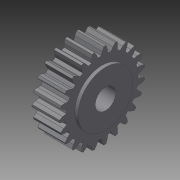
# Autodesk Inventor part: M-0.5 Zb-4mm M-0.7 Zb-5mm mN 21102300
Saved by Autodesk Inventor 2017.3 (Build 213256000, 256)
## iProperties
Category: PARTsolutions
Company: MAEDLER
Created: 2018-08-16
Part Number: M-0.5 Zb-4mm M-0.7 Zb-5mm mN 21102300
Material: Generic
Catalog Web Link: www.cadenas.de
Description: M-0.5 Zb-4mm M-0.7 Zb-5mm mN-Spur Gears, Steel, Module 0.5 and 0,7
Vendor: MAEDLER
Document SubType Name: Modeling
Designer: psadmin
Manufacturer: MAEDLER
Mass: 4 g
Surface Area: 6.38111 cm^2
Volume: 0.554317 cm^3
Density: 1 g/cm^3
Appearance: PSOLRGB-175-175-175
PSOL_IDENT_0: {$CADENAS_DATA\23d-libs\maedler\antriebselemente\stirnzahnraeder\stirnzahnraeder_stahl\modul_0.5_und
PSOL_IDENT_1: _0.7\m-0.5_zb-4mm_m-0.7_zb-5mm_mn.prj},237 {VTYP=3D},{NB=M-0.5 Zb-4mm M-0.7 Zb-5mm mN 21102300},{LIN
PSOL_IDENT_2: A=M-0.5 Zb-4mm M-0.7 Zb-5mm mN 21102300},{NN=M-0.5 Zb-4mm M-0.7 Zb-5mm mN},{DATE=27.10.2015 07:21:56
PSOL_IDENT_3: },{GEOMDATE=11.05.2009 09:51:00},{VERSION=},{LINEID=130},{WBVAR=},{WBNUMERIC=}  {NB=M-0.5 Zb-4mm M-0
PSOL_IDENT_4: .7 Zb-5mm mN 21102300},{LINA=M-0.5 Zb-4mm M-0.7 Zb-5mm mN 21102300},{KT=DUMMY},{ARTNR=21102300},{WST=
PSOL_IDENT_5: 11SMnPb30},{M=0.5},{Z=23},{PDF=PDF Katalogseite},{B1=4.0},{DA=12.50},{D=11.50},{NL=4},{ND=8},{B=3},{
PSOL_IDENT_6: MD=3.0},{GEW=4.000}
NN: M-0.5 Zb-4mm M-0.7 Zb-5mm mN
NT: Spur Gears, Steel, Module 0.5 and 0,7
NB: M-0.5 Zb-4mm M-0.7 Zb-5mm mN 21102300
NBSYN: M-0.5 Zb-4mm M-0.7 Zb-5mm mN $ARTNR.
LINA: M-0.5 Zb-4mm M-0.7 Zb-5mm mN 21102300
ARTNR: 21102300
WST: 11SMnPb30
M: 0.5
Z: 23
PDF: PDF Katalogseite
B1: 4
DA: 12.5
D: 11.5
NL: 4
ND: 8
B: 3
MD: 3
GEW: 4
SUPPLIER: MAEDLER
ARTICLENO: M-0.5 Zb-4mm M-0.7 Zb-5mm mN 21102300
BOMINFO: M-0.5 Zb-4mm M-0.7 Zb-5mm mN 21102300
CREATOR: CADENAS GmbH
Title: M-0.5 Zb-4mm M-0.7 Zb-5mm mN 21102300
Author: Cadenas PARTsolutions
Comments: Spur Gears, Steel, Module 0.5 and 0,7
Autodesk Inventor part; units mm, degrees
ref_plane "YZ Plane" through (0, 0, 0) normal (1, 0, 0) x (0, 1, 0)
ref_plane "XZ Plane" through (0, 0, 0) normal (0, 1, 0) x (-1, 0, 0)
ref_plane "XY Plane" through (0, 0, 0) normal (0, 0, 1) x (1, 0, 0)
sketch "Skizze_1" plane through (0, 0, 0) normal (1, 0, 0) x (0, 1, 0)
  line L0 (0.2601, 6.2446) -> (0.0251, 5.7499)
  line L1 (0.0251, 5.7499) -> (-0.1195, 5.2486)
  arc A0 (-0.1195, 5.2486) -> (-0.5963, 5.216) centre (0, 0) ccw
  line L2 (-0.5963, 5.216) -> (-0.8078, 5.693)
  line L3 (-0.8078, 5.693) -> (-1.108, 6.151)
  arc A1 (-1.108, 6.151) -> (-1.4343, 6.0832) centre (0, 0) ccw
  line L4 (-1.4343, 6.0832) -> (-1.5272, 5.5435)
  line L5 (-1.5272, 5.5435) -> (-1.5311, 5.0218)
  arc A2 (-1.5311, 5.0218) -> (-1.9815, 4.8617) centre (0, 0) ccw
  line L6 (-1.9815, 4.8617) -> (-2.3138, 5.2639)
  line L7 (-2.3138, 5.2639) -> (-2.7264, 5.624)
  arc A3 (-2.7264, 5.624) -> (-3.0224, 5.4706) centre (0, 0) ccw
  line L8 (-3.0224, 5.4706) -> (-2.9662, 4.9259)
  line L9 (-2.9662, 4.9259) -> (-2.8292, 4.4224)
  arc A4 (-2.8292, 4.4224) -> (-3.2197, 4.1468) centre (0, 0) ccw
  line L10 (-3.2197, 4.1468) -> (-3.6482, 4.4445)
  line L11 (-3.6482, 4.4445) -> (-4.1426, 4.6799)
  arc A5 (-4.1426, 4.6799) -> (-4.3862, 4.4523) centre (0, 0) ccw
  line L12 (-4.3862, 4.4523) -> (-4.1852, 3.943)
  line L13 (-4.1852, 3.943) -> (-3.9175, 3.4951)
  arc A6 (-3.9175, 3.4951) -> (-4.2191, 3.1244) centre (0, 0) ccw
  line L14 (-4.2191, 3.1244) -> (-4.712, 3.2954)
  line L15 (-4.712, 3.2954) -> (-5.2516, 3.3886)
  arc A7 (-5.2516, 3.3886) -> (-5.4248, 3.1038) centre (0, 0) ccw
  line L16 (-5.4248, 3.1038) -> (-5.0938, 2.6676)
  line L17 (-5.0938, 2.6676) -> (-4.7152, 2.3086)
  arc A8 (-4.7152, 2.3086) -> (-4.9056, 1.8703) centre (0, 0) ccw
  line L18 (-4.9056, 1.8703) -> (-5.4263, 1.9019)
  line L19 (-5.4263, 1.9019) -> (-5.9711, 1.8461)
  arc A9 (-5.9711, 1.8461) -> (-6.0611, 1.5251) centre (0, 0) ccw
  line L20 (-6.0611, 1.5251) -> (-5.6246, 1.1944)
  line L21 (-5.6246, 1.1944) -> (-5.1632, 0.9509)
  arc A10 (-5.1632, 0.9509) -> (-5.2282, 0.4774) centre (0, 0) ccw
  line L22 (-5.2282, 0.4774) -> (-5.7383, 0.3674)
  line L23 (-5.7383, 0.3674) -> (-6.2478, 0.1667)
  arc A11 (-6.2478, 0.1667) -> (-6.2478, -0.1667) centre (0, 0) ccw
  line L24 (-6.2478, -0.1667) -> (-5.7383, -0.3674)
  line L25 (-5.7383, -0.3674) -> (-5.2282, -0.4774)
  arc A12 (-5.2282, -0.4774) -> (-5.1632, -0.9509) centre (0, 0) ccw
  line L26 (-5.1632, -0.9509) -> (-5.6246, -1.1944)
  line L27 (-5.6246, -1.1944) -> (-6.0611, -1.5251)
  arc A13 (-6.0611, -1.5251) -> (-5.9711, -1.8461) centre (0, 0) ccw
  line L28 (-5.9711, -1.8461) -> (-5.4263, -1.9019)
  line L29 (-5.4263, -1.9019) -> (-4.9056, -1.8703)
  arc A14 (-4.9056, -1.8703) -> (-4.7152, -2.3086) centre (0, 0) ccw
  line L30 (-4.7152, -2.3086) -> (-5.0938, -2.6676)
  line L31 (-5.0938, -2.6676) -> (-5.4248, -3.1038)
  arc A15 (-5.4248, -3.1038) -> (-5.2516, -3.3886) centre (0, 0) ccw
  line L32 (-5.2516, -3.3886) -> (-4.712, -3.2954)
  line L33 (-4.712, -3.2954) -> (-4.2191, -3.1244)
  arc A16 (-4.2191, -3.1244) -> (-3.9175, -3.4951) centre (0, 0) ccw
  line L34 (-3.9175, -3.4951) -> (-4.1852, -3.943)
  line L35 (-4.1852, -3.943) -> (-4.3862, -4.4523)
  arc A17 (-4.3862, -4.4523) -> (-4.1426, -4.6799) centre (0, 0) ccw
  line L36 (-4.1426, -4.6799) -> (-3.6482, -4.4445)
  line L37 (-3.6482, -4.4445) -> (-3.2197, -4.1468)
  arc A18 (-3.2197, -4.1468) -> (-2.8292, -4.4224) centre (0, 0) ccw
  line L38 (-2.8292, -4.4224) -> (-2.9662, -4.9259)
  line L39 (-2.9662, -4.9259) -> (-3.0224, -5.4706)
  arc A19 (-3.0224, -5.4706) -> (-2.7264, -5.624) centre (0, 0) ccw
  line L40 (-2.7264, -5.624) -> (-2.3138, -5.2639)
  line L41 (-2.3138, -5.2639) -> (-1.9815, -4.8617)
  arc A20 (-1.9815, -4.8617) -> (-1.5311, -5.0218) centre (0, 0) ccw
  line L42 (-1.5311, -5.0218) -> (-1.5272, -5.5435)
  line L43 (-1.5272, -5.5435) -> (-1.4343, -6.0832)
  arc A21 (-1.4343, -6.0832) -> (-1.108, -6.151) centre (0, 0) ccw
  line L44 (-1.108, -6.151) -> (-0.8078, -5.693)
  line L45 (-0.8078, -5.693) -> (-0.5963, -5.216)
  arc A22 (-0.5963, -5.216) -> (-0.1195, -5.2486) centre (0, 0) ccw
  line L46 (-0.1195, -5.2486) -> (0.0251, -5.7499)
  line L47 (0.0251, -5.7499) -> (0.2601, -6.2446)
  arc A23 (0.2601, -6.2446) -> (0.5926, -6.2218) centre (0, 0) ccw
  line L48 (0.5926, -6.2218) -> (0.7581, -5.6998)
  line L49 (0.7581, -5.6998) -> (0.8331, -5.1835)
  arc A24 (0.8331, -5.1835) -> (1.301, -5.0862) centre (0, 0) ccw
  line L50 (1.301, -5.0862) -> (1.5755, -5.53)
  line L51 (1.5755, -5.53) -> (1.9352, -5.9428)
  arc A25 (1.9352, -5.9428) -> (2.2493, -5.8312) centre (0, 0) ccw
  line L52 (2.2493, -5.8312) -> (2.2678, -5.2839)
  line L53 (2.2678, -5.2839) -> (2.2007, -4.7665)
  arc A26 (2.2007, -4.7665) -> (2.625, -4.5466) centre (0, 0) ccw
  line L54 (2.625, -4.5466) -> (3.009, -4.8998)
  line L55 (3.009, -4.8998) -> (3.4668, -5.2004)
  arc A27 (3.4668, -5.2004) -> (3.7391, -5.0081) centre (0, 0) ccw
  line L56 (3.7391, -5.0081) -> (3.6093, -4.4761)
  line L57 (3.6093, -4.4761) -> (3.4051, -3.996)
  arc A28 (3.4051, -3.996) -> (3.7543, -3.6698) centre (0, 0) ccw
  line L58 (3.7543, -3.6698) -> (4.2194, -3.9063)
  line L59 (4.2194, -3.9063) -> (4.7413, -4.0722)
  arc A29 (4.7413, -4.0722) -> (4.9517, -3.8136) centre (0, 0) ccw
  line L60 (4.9517, -3.8136) -> (4.6831, -3.3364)
  line L61 (4.6831, -3.3364) -> (4.3569, -2.9292)
  arc A30 (4.3569, -2.9292) -> (4.6052, -2.5208) centre (0, 0) ccw
  line L62 (4.6052, -2.5208) -> (5.1168, -2.6231)
  line L63 (5.1168, -2.6231) -> (5.6641, -2.642)
  arc A31 (5.6641, -2.642) -> (5.7969, -2.3363) centre (0, 0) ccw
  line L64 (5.7969, -2.3363) -> (5.4096, -1.9492)
  line L65 (5.4096, -1.9492) -> (4.9856, -1.6451)
  arc A32 (4.9856, -1.6451) -> (5.1145, -1.1849) centre (0, 0) ccw
  line L66 (5.1145, -1.1849) -> (5.6348, -1.1453)
  line L67 (5.6348, -1.1453) -> (6.1669, -1.0159)
  arc A33 (6.1669, -1.0159) -> (6.2123, -0.6856) centre (0, 0) ccw
  line L68 (6.2123, -0.6856) -> (5.7348, -0.4174)
  line L69 (5.7348, -0.4174) -> (5.2446, -0.239)
  arc A34 (5.2446, -0.239) -> (5.2446, 0.239) centre (0, 0) ccw
  line L70 (5.2446, 0.239) -> (5.7348, 0.4174)
  line L71 (5.7348, 0.4174) -> (6.2123, 0.6856)
  arc A35 (6.2123, 0.6856) -> (6.1669, 1.0159) centre (0, 0) ccw
  line L72 (6.1669, 1.0159) -> (5.6348, 1.1453)
  line L73 (5.6348, 1.1453) -> (5.1145, 1.1849)
  arc A36 (5.1145, 1.1849) -> (4.9856, 1.6451) centre (0, 0) ccw
  line L74 (4.9856, 1.6451) -> (5.4096, 1.9492)
  line L75 (5.4096, 1.9492) -> (5.7969, 2.3363)
  arc A37 (5.7969, 2.3363) -> (5.6641, 2.642) centre (0, 0) ccw
  line L76 (5.6641, 2.642) -> (5.1168, 2.6231)
  line L77 (5.1168, 2.6231) -> (4.6052, 2.5208)
  arc A38 (4.6052, 2.5208) -> (4.3569, 2.9292) centre (0, 0) ccw
  line L78 (4.3569, 2.9292) -> (4.6831, 3.3364)
  line L79 (4.6831, 3.3364) -> (4.9517, 3.8136)
  arc A39 (4.9517, 3.8136) -> (4.7413, 4.0722) centre (0, 0) ccw
  line L80 (4.7413, 4.0722) -> (4.2194, 3.9063)
  line L81 (4.2194, 3.9063) -> (3.7543, 3.6698)
  arc A40 (3.7543, 3.6698) -> (3.4051, 3.996) centre (0, 0) ccw
  line L82 (3.4051, 3.996) -> (3.6093, 4.4761)
  line L83 (3.6093, 4.4761) -> (3.7391, 5.0081)
  arc A41 (3.7391, 5.0081) -> (3.4668, 5.2004) centre (0, 0) ccw
  line L84 (3.4668, 5.2004) -> (3.009, 4.8998)
  line L85 (3.009, 4.8998) -> (2.625, 4.5466)
  arc A42 (2.625, 4.5466) -> (2.2007, 4.7665) centre (0, 0) ccw
  line L86 (2.2007, 4.7665) -> (2.2678, 5.2839)
  line L87 (2.2678, 5.2839) -> (2.2493, 5.8312)
  arc A43 (2.2493, 5.8312) -> (1.9352, 5.9428) centre (0, 0) ccw
  line L88 (1.9352, 5.9428) -> (1.5755, 5.53)
  line L89 (1.5755, 5.53) -> (1.301, 5.0862)
  arc A44 (1.301, 5.0862) -> (0.8331, 5.1835) centre (0, 0) ccw
  line L90 (0.8331, 5.1835) -> (0.7581, 5.6998)
  line L91 (0.7581, 5.6998) -> (0.5926, 6.2218)
  arc A45 (0.5926, 6.2218) -> (0.2601, 6.2446) centre (0, 0) ccw
  constraints: 184 end point, 92 point on circle, 46 centre point
extrude "Extrusion1" add sketch "Skizze_1" along normal mid plane 4
sketch "Skizze_2" plane through (0, 0, 0) normal (0, 0, 1) x (1, 0, 0)
  line L0 (6, 0) -> (2, 0)
  line L1 (2, 0) -> (2, 4)
  line L2 (2, 4) -> (6, 4)
  line L3 (6, 4) -> (6, 0)
  line L4 (6, 0) -> (2, 0)
  constraints: 10 end point
revolve "Revolution1" add sketch "Skizze_2" angle 360 about axis through (6, 0, 0) along (1, 0, 0)
sketch "Skizze_3" plane through (6, 0, 0) normal (1, 0, 0) x (0, 1, 0)
  circle A0 centre (0, 0) radius 1.5
  constraints: 1 centre point
extrude "Extrusion2" cut sketch "Skizze_3" along normal mid plane 16
sketch "Skizze4" plane through (6, 0, 0) normal (1, 0, 0) x (0, 0, -1)
  circle A0 centre (0, 0) radius 4 projected
extrude "Extrusion3" cut sketch "Skizze4" against normal blind 3.5
body "Solid1"
